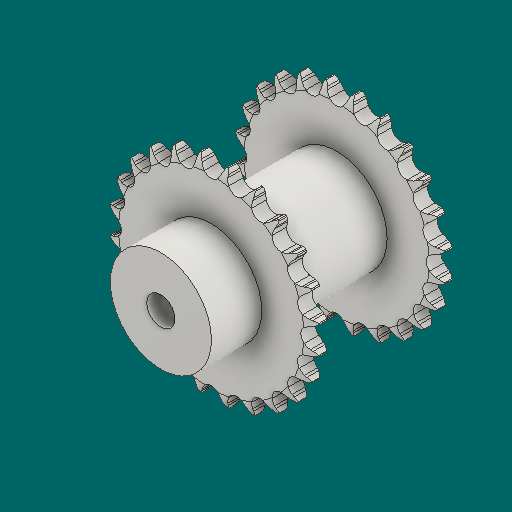
# Autodesk Inventor part: Roller Chain Sprocket1
Saved by Autodesk Inventor 2023 (Build 270158000, 158)
## iProperties
CustomPartVersion: 1
Created: 2023-01-28
Part Number: Roller Chain Sprocket1
Material: Steel
Document SubType Name: Modeling
Designer: HeavyDrewno
Density: 1 g/cm^3
Appearance: Steel
d28: 0,000 mm
d29: 0,000 mm
d42: 0,000 mm
Author: HeavyDrewno
Autodesk Inventor part; units mm, degrees
ref_plane "YZ Plane" through (0, 0, 0) normal (1, 0, 0) x (0, 1, 0)
ref_plane "XZ Plane" through (0, 0, 0) normal (0, 1, 0) x (-1, 0, 0)
sketch "Theoretical Tooth Profile" plane through (0, 0, 0) normal (0, 0, 1) x (1, 0, 0)
  circle A0 centre (0, 0) radius 48.6492 construction
  line L0 (0, 0) -> (0, 48.6492) construction
  line L1 (0, 0) -> (12.5913, 46.9916) construction
  circle A1 centre (0, 0) radius 52.043
  arc A2 (-3.4095, 46.0331) -> (3.4095, 46.0331) centre (0, 48.6492) ccw
  line L2 (0, 48.6492) -> (12.5913, 46.9916) construction
  line L3 (0, 48.6492) -> (5.4011, 52.7937) construction
  line L4 (5.4011, 52.7937) -> (-4.9078, 48.6634) construction
  arc A3 (6.4953, 51.6361) -> (5.321, 49.6948) centre (11.8121, 47.0942) ccw
  arc A4 (-5.321, 49.6948) -> (-6.4953, 51.6361) centre (-11.8121, 47.0942) ccw
  line L5 (-11.8121, 47.0942) -> (-5.321, 49.6948) construction
  arc A5 (-4.9078, 48.6634) -> (-3.4095, 46.0331) centre (5.4011, 52.7937) ccw
  line L6 (-4.9078, 48.6634) -> (-5.321, 49.6948)
  arc A6 (3.4095, 46.0331) -> (4.9078, 48.6634) centre (-5.4011, 52.7937) ccw
  line L7 (5.321, 49.6948) -> (4.9078, 48.6634)
  line L8 (0, 0) -> (6.793, 51.5978) construction
  point P0 (6.2957, 47.8204)
  dimension "d0" = 97.2985
  dimension "d2" = 15
  dimension "d3" = 4.2976
  dimension "d10" = 127.5
  dimension "d11" = 15.667
  dimension "d12" = 6.808
  dimension "d13" = 11.1055
  dimension "d14" = 11.914
  dimension "d23" = 3.81
  constraints: 18 end point, 15 point on circle, 7 centre point, 3 coincident, 3 point on line, 3 symmetric about line, 3 tangent, 1 equal radius, 1 midpoint, 1 parallel, 1 vertical, 1 other
  measures "d0" diameter of A0
  measures "d2" angle of L1 L0
  measures "d3" radius of A2
  measures "d10" angle of L3 L0
  measures "d11" angle of L4 L3
  measures "d12" distance of L2.start L3.end
  measures "d13" distance of L3.end L4.end
  measures "d14" distance of A3.centre L0.end
  measures "d23" distance from line of L8.end L2
sketch "Tooth Profile" plane through (0, 0, 0) normal (0, 0, 1) x (1, 0, 0)
  arc A0 (-3.9881, 47.048) -> (3.9881, 47.048) centre (0, 48.6492) ccw
  arc A1 (6.382, 51.6503) -> (3.9881, 47.048) centre (28.6276, 37.1555) ccw
  arc A2 (-3.9881, 47.048) -> (-6.382, 51.6503) centre (-28.6276, 37.1555) ccw
  line L0 (0, 0) -> (0, 48.6492) construction
  line L1 (0, 48.6492) -> (3.9881, 47.048) construction
  line L2 (0, 48.6492) -> (-3.9881, 47.048) construction
  circle A3 centre (0, 0) radius 52.043 projected
  dimension "d44" = 136.25
  dimension "d45" = 26.5512
  dimension "d46" = 4.2976
  constraints: 9 point on circle, 6 end point, 3 centre point, 2 tangent, 1 coincident, 1 equal radius, 1 vertical, 1 other
  measures "d44" angle of L2 L1
  measures "d45" radius of A1
  measures "d46" radius of A0
sketch "Section Profile" plane through (0, 0, 0) normal (1, 0, 0) x (0, 1, 0)
  line L0 (52.043, 0) -> (-52.043, 0) projected
  line L1 (37.7838, 3.6038) -> (-37.7838, 3.6038)
  line L2 (-37.7838, 3.6038) -> (-37.7838, -3.6037)
  line L3 (-37.7838, -3.6037) -> (37.7838, -3.6037)
  line L4 (37.7838, -3.6037) -> (37.7838, 3.6038)
  line L5 (37.7838, 3.6037) -> (52.043, 3.6037) construction
  line L6 (52.043, 3.6037) -> (52.043, -3.6037) construction
  line L7 (52.043, -3.6037) -> (37.7838, -3.6037) construction
  line L8 (37.7838, -3.6037) -> (37.7838, 3.6037)
  arc A0 (52.043, 1.9527) -> (45.7813, 3.6037) centre (45.7813, -9.0962) ccw
  arc A1 (45.7813, -3.6037) -> (52.043, -1.9527) centre (45.7813, 9.0962) ccw
  line L9 (45.7813, 3.6037) -> (0, 3.6037)
  line L10 (0, 3.6037) -> (0, -3.6037)
  line L11 (0, -3.6037) -> (45.7813, -3.6037)
  line L12 (0, 3.6037) -> (0, -3.6037)
  line L13 (52.043, 1.9527) -> (52.043, -1.9527)
  point P0 (0, 0)
  point P1 (0, 0)
  dimension "d30" = 7.2075
  dimension "d31" = 75.5677
  dimension "d32" = 7.2075
  dimension "d33" = 1.651
  dimension "d34" = 12.7
  dimension "d43" = 3.6037
  constraints: 26 end point, 7 midpoint, 5 perpendicular, 4 parallel, 4 point on circle, 3 point on line, 3 symmetric about line, 2 centre point, 2 horizontal, 2 tangent, 1 collinear, 1 other
  measures "d30" distance between parallel lines of L7 L5
  measures "d31" distance between parallel lines of L2 L4
  measures "d32" distance between parallel lines of L3 L1
  measures "d33" distance from line of L13.start L5
  measures "d34" radius of A0
  measures "d43" distance between parallel lines of L3 L0
revolve "Shroud" add sketch "Section Profile" angle 360 about axis through (0, 0, 3.6037) along (0, 0, -1) contours L10 L3 L2 L0 | L0 L2 L1 L10
revolve "Strand" add sketch "Section Profile" angle 360 about axis through (0, 0, 3.6037) along (0, 0, -1) contours L13 A1 L11 L4 L0 | L0 L4 L9 A0 L13 | L4 L3 L10 L0 | L0 L10 L1 L4
pattern_of_one "Strand Pattern"
extrude "Theoretical Tooth" cut sketch "Theoretical Tooth Profile" along normal through all both and the other way through all contours A3 L7 A6 A2 A5 L6 A4 A1 picked at (0, 49.449)
extrude "Tooth" [suppressed]
pattern_circular "Tooth Pattern" count 24 over 360 about axis through (0, 0, -10) along (0, 0, 1) of "Theoretical Tooth"
ref_plane "Timing Plane" through (0, 48.6492, 0) normal (1, 0, 0) x (0, 1, 0)
sketch "Sketch4" plane through (0, 48.6492, 3.6038) normal (0, 0, 1) x (1, 0, 0)
  circle A0 centre (0, -48.6492) radius 25
  dimension "d51" = 50
  constraints: 1 centre point, 1 coincident
  measures "d51" diameter of A0
extrude "Extrusion4" add sketch "Sketch4" along normal blind 27.4
mirror "Mirror1" about plane through (0, 0, 31.0038) normal (0, 0, 1)
sketch "Sketch5" plane through (0, 48.6492, 65.6113) normal (0, 0, 1) x (1, 0, 0)
  circle A0 centre (0, -48.6492) radius 25
  constraints: 1 centre point, 1 coincident
extrude "Extrusion5" add sketch "Sketch5" along normal blind 24.9
sketch "Sketch6" plane through (0, 48.6492, -3.6037) normal (0, 0, -1) x (-1, 0, 0)
  point P0 (0, -48.6492)
  point P1 (0, -48.6492)
  constraints: 1 coincident
hole "Hole1" at (0, 0, -3.6037) direction (0, 0, 1) diameter 14 end through all
equation "\"d3\" = 0.5 * da_Dr + da_SC"
equation "\"d12\" = 0.8 * da_Dr"
equation "\"d13\" = 1.3 * da_Dr + da_SC"
equation "\"d14\" = 1.4 * da_Dr"
equation "\"d23\" = da_Ha"
equation "\"d44\" = da_Alfa"
equation "\"d45\" = da_Re"
equation "\"d46\" = da_Ri"
equation "\"d30\" = da_Bf"
equation "\"d31\" = da_Ds"
equation "\"d32\" = da_Bs"
equation "\"d33\" = da_Ba"
equation "\"d34\" = da_Rx"
equation "\"d40\" = da_pt"
equation "\"form_type\" = 0"
equation "\"da_p\" = 12.7"
equation "\"da_Dr\" = 8.51"
equation "\"da_SC\" = 0.04255"
equation "\"da_Ha\" = 3.81"
equation "\"da_pt\" = 13.92"
equation "\"da_Bf\" = 7.2075"
equation "\"da_Ba\" = 1.651"
equation "\"da_Rx\" = 12.7"
equation "\"da_Ra\" = 0.508"
equation "\"da_Bs\" = 7.2075"
equation "\"da_Ds\" = 75.56768"
equation "\"da_Re\" = 26.5512"
equation "\"da_Ri\" = 4.29755"
equation "\"da_Alfa\" = 136.25deg"
body "Solid1"
